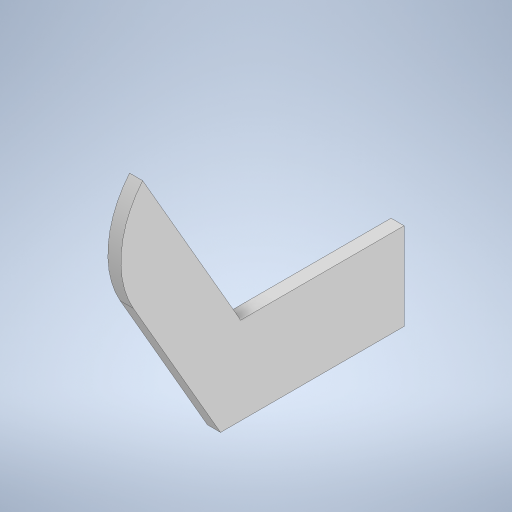
# Autodesk Inventor part: claw2
Saved by Autodesk Inventor 2024.1 (Build 281209000, 209)
## iProperties
Created: 2024-02-14
Part Number: claw2
Material: 一般
Document SubType Name: Modeling
Designer: hibik
Density: 1 g/cm^3
Appearance: 既定
Author: hibik
Autodesk Inventor part; units mm, degrees
ref_plane "YZ Plane" through (0, 0, 0) normal (1, 0, 0) x (0, 1, 0)
ref_plane "XZ Plane" through (0, 0, 0) normal (0, 1, 0) x (-1, 0, 0)
ref_plane "XY Plane" through (0, 0, 0) normal (0, 0, 1) x (1, 0, 0)
sketch "スケッチ1" plane through (0, 0, 0) normal (1, 0, 0) x (0, 1, 0)
  line L0 (10, 0) -> (0, 0)
  line L1 (0, 0) -> (0, -15)
  line L2 (0, -15) -> (10, -15)
  line L3 (10, -15) -> (10, 0)
  line L4 (10, 0) -> (0, 0)
  line L5 (0, 0) -> (0, 6.0622)
  line L6 (0, 6.0622) -> (10, 6.0622)
  line L7 (10, 6.0622) -> (10, 0)
  line L8 (0, 6.0622) -> (3.5, 0)
  line L9 (3.5, 0) -> (29.4808, 15)
  line L10 (29.4808, 15) -> (25.9808, 21.0622)
  line L11 (25.9808, 21.0622) -> (0, 6.0622)
  arc A0 (29.4808, 15) -> (17.3205, 16.0622) centre (22.6419, 6.8452) ccw
  point P0 (10, 3.7528)
  dimension "d0" = 10
  dimension "d1" = 15
  dimension "d6" = 30
  dimension "d10" = 60
  dimension "d11" = 7
  dimension "d12" = 20
  constraints: 24 end point, 6 parallel, 3 perpendicular, 2 horizontal, 2 point on circle, 2 point on line, 1 centre point, 1 coincident, 1 collinear, 1 tangent
  measures "d0" distance of L0.start L0.end
  measures "d1" distance of L2.end L0.start
  measures "d6" distance between parallel lines of L10 L8
  measures "d10" angle of L7 L9
  measures "d11" distance between parallel lines of L9 L11
  measures "d12" distance from line of L8 A0.end
extrude "押し出し1" add sketch "スケッチ1" along normal blind 1.5 contours L3 L2 L1 L0 | L0 L9 L7 | L0 L5 L8 | L8 L6 L7 L9 | L7 L6 L11 A0 L9
